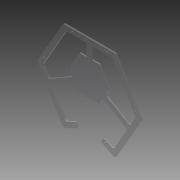
# Autodesk Inventor part: Top Plat
Saved by Autodesk Inventor 2015 (Build 190159000, 159)
## iProperties
Created: 2016-10-14
Part Number: Top Plat
Material: Polycarbonate, Clear
Document SubType Name: Modeling
Designer: James Yelland
Density: 1.2 g/cm^3
Appearance: Polycarbonate - Clear
Author: James Yelland
Autodesk Inventor part; units mm, degrees
ref_plane "YZ Plane" through (0, 0, 0) normal (1, 0, 0) x (0, 1, 0)
ref_plane "XZ Plane" through (0, 0, 0) normal (0, 1, 0) x (-1, 0, 0)
ref_plane "XY Plane" through (0, 0, 0) normal (0, 0, 1) x (1, 0, 0)
sketch "Sketch1" plane through (0, 0, 0) normal (0, 1, 0) x (-1, 0, 0)
  circle A0 centre (30.6147, -73.9104) radius 1.6
  circle A1 centre (-30.6147, -73.9104) radius 1.6
  circle A2 centre (30.6147, -73.9104) radius 1.6
  circle A3 centre (-30.6147, -73.9104) radius 1.6
  line L0 (103.5566, -2.5) -> (54.8095, -86.9325)
  line L1 (-54.8095, -86.9325) -> (-103.5566, -2.5)
  line L2 (-103.5566, 2.5) -> (-53.9434, 88.4327)
  line L3 (-49.6132, 90.9327) -> (49.6132, 90.9327)
  line L4 (53.9434, 88.4327) -> (103.5566, 2.5)
  arc A4 (48.3297, -88.9468) -> (54.8095, -86.9325) centre (50.4794, -84.4325) ccw
  arc A5 (-54.8095, -86.9325) -> (-48.3297, -88.9468) centre (-50.4794, -84.4325) ccw
  arc A6 (-103.5566, 2.5) -> (-103.5566, -2.5) centre (-99.2265, 0) ccw
  arc A7 (-49.6132, 90.9327) -> (-53.9434, 88.4327) centre (-49.6132, 85.9327) ccw
  arc A8 (53.9434, 88.4327) -> (49.6132, 90.9327) centre (49.6132, 85.9327) ccw
  arc A9 (103.5566, -2.5) -> (103.5566, 2.5) centre (99.2265, 0) ccw
  line L5 (-92.0094, 2.5) -> (-48.1698, 78.4325)
  line L6 (48.1698, 78.4325) -> (92.0094, 2.5)
  arc A10 (-43.8396, 80.9325) -> (-48.1698, 78.4325) centre (-43.8396, 75.9325) ccw
  arc A11 (-92.0094, 2.5) -> (-92.0094, -2.5) centre (-87.6793, 0) ccw
  line L7 (32.3518, -70.2624) -> (44.2883, -75.9464)
  arc A12 (44.2883, -75.9464) -> (50.7681, -73.9321) centre (46.4379, -71.4321) ccw
  line L8 (32.3518, -70.2624) -> (29.6432, -68.9726)
  line L9 (26.9776, -69.9184) -> (24.398, -75.3356)
  arc A13 (29.6432, -68.9726) -> (26.9776, -69.9184) centre (28.7834, -70.7783) ccw
  arc A14 (24.398, -75.3356) -> (25.3439, -78.0012) centre (26.2038, -76.1955) ccw
  circle A15 centre (-30.6147, -73.9104) radius 1.6
  circle A16 centre (-30.6147, -73.9104) radius 1.6
  line L10 (-32.3518, -70.2624) -> (-44.2883, -75.9464)
  arc A17 (-50.7681, -73.9321) -> (-44.2883, -75.9464) centre (-46.4379, -71.4321) ccw
  line L11 (-32.3518, -70.2624) -> (-29.6432, -68.9726)
  line L12 (-26.9776, -69.9184) -> (-24.398, -75.3356)
  arc A18 (-26.9776, -69.9184) -> (-29.6432, -68.9726) centre (-28.7834, -70.7783) ccw
  arc A19 (-25.3439, -78.0012) -> (-24.398, -75.3356) centre (-26.2038, -76.1955) ccw
  line L13 (48.3297, -88.9468) -> (25.3439, -78.0012)
  line L14 (-25.3439, -78.0012) -> (-48.3297, -88.9468)
  line L15 (-70.0896, 40.4662) -> (-67.5896, 44.7964)
  line L16 (-70.0896, 40.4662) -> (-72.5896, 36.1361)
  line L17 (-5, 77.9325) -> (-5, 58.9325)
  line L18 (-8, 55.9325) -> (-18.2679, 55.9325)
  line L19 (-20.866, 54.4325) -> (-39.134, 22.7915)
  line L20 (-18.2679, -13.3495) -> (18.2679, -13.3495)
  line L21 (20.866, -11.8495) -> (26, -2.9572)
  line L22 (30.0981, -1.8592) -> (74.211, -27.3278)
  line L23 (-20.866, -11.8495) -> (-26, -2.9572)
  line L24 (-30.0981, -1.8592) -> (-74.211, -27.3278)
  line L25 (-39.134, 19.7915) -> (-34, 10.8992)
  line L26 (-35.0981, 6.8011) -> (-79.211, -18.6675)
  arc A20 (18.2679, -13.3495) -> (20.866, -11.8495) centre (18.2679, -10.3495) ccw
  arc A21 (-20.866, -11.8495) -> (-18.2679, -13.3495) centre (-18.2679, -10.3495) ccw
  arc A22 (-39.134, 22.7915) -> (-39.134, 19.7915) centre (-36.5359, 21.2915) ccw
  arc A23 (-18.2679, 55.9325) -> (-20.866, 54.4325) centre (-18.2679, 52.9325) ccw
  arc A24 (-8, 55.9325) -> (-5, 58.9325) centre (-8, 58.9325) ccw
  arc A25 (30.0981, -1.8592) -> (26, -2.9572) centre (28.5981, -4.4572) ccw
  line L27 (-8, 80.9325) -> (-43.8396, 80.9325)
  line L28 (75.3091, -31.4258) -> (50.7681, -73.9321)
  line L29 (-50.7681, -73.9321) -> (-75.3091, -31.4258)
  line L30 (-83.3091, -17.5694) -> (-92.0094, -2.5)
  arc A26 (75.3091, -31.4258) -> (74.211, -27.3278) centre (72.711, -29.9258) ccw
  arc A27 (-74.211, -27.3278) -> (-75.3091, -31.4258) centre (-72.711, -29.9258) ccw
  arc A28 (-83.3091, -17.5694) -> (-79.211, -18.6675) centre (-80.711, -16.0694) ccw
  arc A29 (-5, 77.9325) -> (-8, 80.9325) centre (-8, 77.9325) ccw
  line L31 (48.1698, 78.4325) -> (92.0094, 2.5)
  line L32 (48.1698, 78.4325) -> (92.0094, 2.5)
  line L33 (5, 77.9325) -> (5, 58.9325)
  line L34 (8, 55.9325) -> (18.2679, 55.9325)
  line L35 (20.866, 54.4325) -> (39.134, 22.7915)
  line L36 (39.134, 19.7915) -> (34, 10.8992)
  line L37 (35.0981, 6.8011) -> (79.211, -18.6675)
  line L38 (83.3091, -17.5694) -> (92.0094, -2.5)
  line L39 (8, 80.9325) -> (43.8396, 80.9325)
  arc A30 (79.211, -18.6675) -> (83.3091, -17.5694) centre (80.711, -16.0694) ccw
  arc A31 (34, 10.8992) -> (35.0981, 6.8011) centre (36.5981, 9.3992) ccw
  arc A32 (39.134, 19.7915) -> (39.134, 22.7915) centre (36.5359, 21.2915) ccw
  arc A33 (20.866, 54.4325) -> (18.2679, 55.9325) centre (18.2679, 52.9325) ccw
  arc A34 (5, 58.9325) -> (8, 55.9325) centre (8, 58.9325) ccw
  arc A35 (8, 80.9325) -> (5, 77.9325) centre (8, 77.9325) ccw
  arc A36 (48.1698, 78.4325) -> (43.8396, 80.9325) centre (43.8396, 75.9325) ccw
  arc A37 (92.0094, -2.5) -> (92.0094, 2.5) centre (87.6793, 0) ccw
  circle A38 centre (35.5991, 85.9437) radius 1.6
  circle A39 centre (-35.5945, 85.9327) radius 1.6
  circle A40 centre (92.2171, 12.1406) radius 1.6
  circle A41 centre (-92.2171, 12.1406) radius 1.6
  arc A42 (-35.0981, 6.8011) -> (-34, 10.8992) centre (-36.5981, 9.3992) ccw
  arc A43 (-26, -2.9572) -> (-30.0981, -1.8592) centre (-28.5981, -4.4572) ccw
  point P0 (105, 0)
  point P1 (52.5, -90.9327)
  point P2 (-105, 0)
  point P3 (-52.5, 90.9327)
  point P4 (52.5, 90.9327)
  point P5 (-93.4528, 0)
  point P6 (-46.7264, 80.9325)
  point P7 (46.7264, 80.9325)
  point P8 (93.4528, 0)
  point P9 (-5, -80.9325)
  point P10 (5, -80.9325)
  point P11 (-5, 55.9325)
  point P12 (-20, 55.9325)
  point P13 (-40, 21.2915)
  point P14 (-20, -13.3495)
  point P15 (20, -13.3495)
  point P16 (-27.5, -0.3592)
  point P17 (-32.5, 8.3011)
  point P18 (5, 80.9325)
  point P19 (5, 55.9325)
  point P20 (20, 55.9325)
  point P21 (40, 21.2915)
  point P22 (32.5, 8.3011)
  dimension "d148" = 5
  dimension "d150" = 2
  dimension "d175" = 40
  dimension "d177" = 40
  dimension "d179" = 40
  dimension "d186" = 15
  dimension "d187" = 15
  dimension "d188" = 3
  dimension "d192" = 25
  dimension "d193" = 15
  dimension "d194" = 40
  dimension "d196" = 15
  dimension "d197" = 90
  dimension "d198" = 3
  dimension "d199" = 5
  constraints: 80 end point, 68 point on circle, 44 centre point, 43 point on line, 20 tangent, 7 equal radius, 3 coincident, 1 horizontal, 1 midpoint, 1 perpendicular
  measures "d148" radius of A12
  measures "d150" radius of A13
  measures "d175" distance of point (-20, 55.932) point (-40, 21.291)
  measures "d177" distance of point (-40, 21.291) point (-20, -13.35)
  measures "d179" distance of point (-20, -13.35) point (20, -13.35)
  measures "d186" distance of point (-20, -13.35) point (-27.5, -0.359)
  measures "d187" distance of point (-40, 21.291) point (-32.5, 8.301)
  measures "d188" radius of A20
  measures "d192" distance of point (5, 80.932) point (5, 55.932)
  measures "d193" distance of point (5, 55.932) point (20, 55.932)
  measures "d194" distance of point (20, 55.932) point (40, 21.291)
  measures "d196" distance of point (40, 21.291) point (32.5, 8.301)
  measures "d197" angle of L37 L36
  measures "d198" radius of A30
  measures "d199" radius of A36
extrude "Extrusion2" add sketch "Sketch1" along normal blind 3
body "Solid2"
